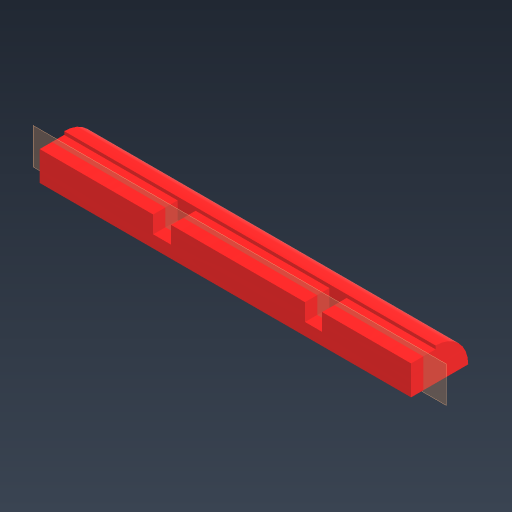
# Autodesk Inventor part: Край задней части корпуса
Saved by Autodesk Inventor 2023.2 (Build 272271030, 271C)
## iProperties
Created: 2025-04-24
Part Number: Край задней части корпуса
Material: Типовые
Document SubType Name: Modeling
Designer: Коноваленко
Density: 1 g/cm^3
Appearance: Светло-красный
Author: Коноваленко
Autodesk Inventor part; units mm, degrees
ref_plane "YZ Plane" through (0, 0, 0) normal (1, 0, 0) x (0, 1, 0)
ref_plane "XZ Plane" through (0, 0, 0) normal (0, 1, 0) x (-1, 0, 0)
ref_plane "XY Plane" through (0, 0, 0) normal (0, 0, 1) x (1, 0, 0)
sketch "Эскиз1" plane through (0, 0, 0) normal (1, 0, 0) x (0, 1, 0)
  line L0 (-8.3221, -24.9171) -> (-8.3221, 15.0829)
  line L1 (-8.3221, 15.0829) -> (31.6779, 15.0829)
  arc A0 (-8.3221, -24.9171) -> (31.6779, 15.0829) centre (-8.3221, 15.0829) ccw
  point P0 (0, 0)
  dimension "d1" = 40
  constraints: 4 end point, 2 line through centre, 2 point on circle, 1 centre point, 1 horizontal, 1 vertical
  measures "d1" distance of L0.end L1.end
extrude "Выдавливание1" add sketch "Эскиз1" along normal mid plane 455
sketch "Эскиз3" plane through (-227.5, -8.3221, 15.0829) normal (0, 0, 1) x (1, 0, 0)
  line L0 (0, 0) -> (455, 0) projected
  line L1 (455, 40) -> (455, 0) projected
  line L2 (455, 40) -> (0, 40) projected
  line L3 (0, 0) -> (0, 40) projected
  point P0 (227.5, 8.3221)
extrude "Выдавливание2" add sketch "Эскиз3" along normal blind 30
sketch "Эскиз4" plane through (-227.5, 31.6779, 15.0829) normal (0, 1, 0) x (1, 0, 0)
  line L0 (455, 0) -> (0, 0) projected
  line L1 (0, 0) -> (0, -30) projected
  line L2 (455, -30) -> (0, -30) projected
  line L3 (455, 0) -> (455, -30) projected
  point P0 (227.5, 15.0829)
extrude "Выдавливание3" cut sketch "Эскиз4" against normal blind 4
sketch "Эскиз6" plane through (-227.5, 27.6779, 15.0829) normal (0, 1, 0) x (1, 0, 0)
  line L0 (0, 40) -> (0, -30) projected
  line L1 (0, -14.536) -> (200.0528, -14.536) construction
  line L2 (455, 0) -> (0, 0) projected
  circle A0 centre (10.061, -14.536) radius 8.0645
  circle A1 centre (37.061, -14.536) radius 8.0645
  circle A2 centre (64.061, -14.536) radius 8.0645
  circle A3 centre (91.061, -14.536) radius 8.0645
  circle A4 centre (118.061, -14.536) radius 8.0645
  circle A5 centre (145.061, -14.536) radius 8.0645
  circle A6 centre (172.061, -14.536) radius 8.0645
  point P0 (227.5, 15.0829)
  dimension "d21" = 14.536
  dimension "d22" = 16.129
  dimension "d23" = 10.061
  dimension "d26" = 27
  constraints: 7 centre point, 2 end point, 2 horizontal, 2 point on line, 12 other
  measures "d21" distance between parallel lines of L2 L1
  measures "d22" diameter of A0
  measures "d23" distance from line of L0 A0.centre
  measures "d26" distance of A0.centre A1.centre
extrude "Выдавливание5" [suppressed]
sketch "Эскиз8" plane through (-227.5, -8.3221, -24.9171) normal (0, -1, 0) x (1, 0, 0)
  line L0 (455, 50) -> (465, 55)
  line L1 (465, 55) -> (465, 35)
  line L2 (465, 35) -> (455, 40)
  line L3 (455, 0) -> (455, 70) projected
  point P0 (227.5, 24.9171)
  point P1 (465, 45)
  dimension "d33" = 20
  dimension "d34" = 10
  dimension "d35" = 20
  dimension "d36" = 15
  dimension "d37" = 10
  constraints: 6 end point, 2 point on line, 1 midpoint, 1 vertical
  measures "d33" distance of L0.end L1.end
  measures "d34" distance of L2.end L0.start
  measures "d35" distance of L3.end L0.start
  measures "d36" vertical distance of L3.end L0.end
  measures "d37" distance from line of point (465, 45) L3
extrude "Выдавливание6" [suppressed]
sketch "Эскиз9" plane through (-227.5, -8.3221, -24.9171) normal (0, -1, 0) x (1, 0, 0)
  line L0 (210, 40) -> (220, 45)
  line L1 (220, 45) -> (220, 25)
  line L2 (220, 25) -> (210, 30)
  line L3 (455, 0) -> (455, 70) projected
  line L4 (-10, 25) -> (-10, 45)
  line L5 (-10, 45) -> (0, 40)
  line L6 (0, 30) -> (-10, 25)
  line L7 (0, 0) -> (0, 70) projected
  point P0 (227.5, 24.9171)
  constraints: 12 end point, 2 vertical, 13 other
extrude "Выдавливание7" [suppressed]
sketch "Эскиз10" plane through (-227.5, -8.3221, -24.9171) normal (0, -1, 0) x (1, 0, 0)
  line L0 (-10, 45) -> (0, 40)
  line L1 (-10, 25) -> (-10, 45)
  line L2 (0, 30) -> (-10, 25)
  line L3 (0, 0) -> (0, 70) projected
  point P0 (227.5, 24.9171)
  constraints: 6 end point, 1 vertical, 6 other
extrude "Выдавливание8" add sketch "Эскиз10" against normal blind 20
sketch "Эскиз11" plane through (-227.5, -8.3221, -24.9171) normal (0, -1, 0) x (1, 0, 0)
  line L0 (0, 70) -> (455, 70) projected
  line L1 (0, 0) -> (455, 0) projected
  line L2 (0, 40) -> (455, 40) projected
  point P0 (227.5, 24.9171)
feature "Разделение1" [suppressed]
sketch "Эскиз14" plane through (-227.5, 27.6779, 15.0829) normal (0, 1, 0) x (1, 0, 0)
  line L0 (0, 0) -> (455, 0) projected
  line L1 (0, -30) -> (455, -30) projected
  line L2 (134.048, 0) -> (100.336, 0)
  line L3 (100.336, 0) -> (100.336, -30) construction
  line L4 (100.336, -30) -> (134.048, -30)
  line L5 (134.048, -30) -> (134.048, 0)
  line L6 (105, 0) -> (105, -320)
  line L7 (319.048, 0) -> (285.336, 0)
  line L8 (285.336, -30) -> (319.048, -30)
  line L9 (319.048, -30) -> (319.048, 0)
  line L10 (290, 0) -> (290, -320)
  point P0 (227.5, 15.0829)
  point P1 (105, -30)
  point P2 (134.048, -30)
  point P3 (290, -30)
  point P4 (319.048, -30)
  dimension "d71" = 33.712
  dimension "d72" = 4.664
  dimension "d75" = 185
  constraints: 18 end point, 2 horizontal, 2 parallel, 2 point on line, 1 perpendicular, 1 vertical, 12 other
  measures "d71" distance between parallel lines of L3 L5
  measures "d72" distance between parallel lines of L3 L6
  measures "d75" distance of L2.start L7.start
extrude "Выдавливание10" [suppressed]
ref_plane "РабПлоскость1" through (-227.5, 31.6779, 30.0829) normal (0, 0, 1) x (1, 0, 0)
sketch "Эскиз16" plane through (-227.5, -8.3221, -24.9171) normal (0, -1, 0) x (1, 0, 0)
  circle A0 centre (115, 55) radius 2.529
  line L0 (-91, 55) -> (546, 55) construction
  line L1 (115, 360) -> (115, 40) construction
  line L2 (300, 360) -> (300, 40) construction
  circle A1 centre (300, 55) radius 2.529
  point P0 (227.5, 24.9171)
  dimension "d82" = 5.058
  constraints: 4 end point, 4 point on line, 2 centre point, 2 vertical, 1 equal radius, 4 other
  measures "d82" diameter of A0
extrude "Выдавливание11" [suppressed]
sketch "Эскиз12" plane through (-227.5, 27.6779, 15.0829) normal (0, 1, 0) x (1, 0, 0)
  line L0 (0, 0) -> (455, 0) projected
  line L1 (248.041, 0) -> (248.041, -5)
  line L2 (248.041, -5) -> (264.217, -4.95)
  line L3 (264.217, -4.95) -> (264.217, -17.926)
  line L4 (264.217, -17.926) -> (248.041, -20.945)
  line L5 (248.041, -20.945) -> (248.041, -30)
  line L6 (0, -30) -> (455, -30) projected
  line L7 (227.5, 54) -> (227.5, -44) projected
  point P0 (227.5, 15.0829)
  dimension "d54" = 20.541
  dimension "d55" = 16.176
  dimension "d56" = 12.074
  dimension "d57" = 4.95
  dimension "d58" = 9.055
  dimension "d59" = 5
  constraints: 10 end point, 4 point on line, 1 parallel, 1 perpendicular
  measures "d54" distance between parallel lines of L7 L5
  measures "d55" distance between parallel lines of L1 L3
  measures "d56" distance from line of L6 L3.end
  measures "d57" distance from line of L0 L2.end
  measures "d58" distance of L4.end L5.end
  measures "d59" distance of L1.start L1.end
feature "Разделение2" [suppressed]
sketch "Эскиз13" plane through (-227.5, 27.6779, 15.0829) normal (0, 1, 0) x (1, 0, 0)
  line L0 (0, -30) -> (455, -30) projected
  line L1 (0, 0) -> (455, 0) projected
  line L2 (346, -30) -> (324, -30)
  line L3 (324, -30) -> (324, 0)
  line L4 (324, 0) -> (346, 0)
  line L5 (346, 0) -> (346, -30)
  line L6 (325, -320) -> (325, 0)
  line L7 (161, -30) -> (139, -30)
  line L8 (139, -30) -> (139, 0)
  line L9 (139, 0) -> (161, 0)
  line L10 (161, 0) -> (161, -30)
  point P0 (227.5, 15.0829)
  point P1 (325, -30)
  point P2 (346, 0)
  point P3 (161, 0)
  dimension "d60" = 22
  dimension "d61" = 1
  dimension "d66" = 185
  constraints: 18 end point, 2 horizontal, 2 parallel, 2 point on line, 1 perpendicular, 1 vertical, 10 other
  measures "d60" distance between parallel lines of L3 L5
  measures "d61" distance between parallel lines of L3 L6
  measures "d66" distance of L2.start L7.start
extrude "Выдавливание9" cut sketch "Эскиз13" against normal blind 21 contours L8 L1 L10 L0 | L6 L1 L5 L0
sketch "Эскиз17" plane through (-227.5, -8.3221, -24.9171) normal (0, -1, 0) x (1, 0, 0)
  circle A0 centre (150, 55) radius 2.1
  line L0 (-91, 55) -> (546, 55) construction
  line L1 (150, 40) -> (150, 360) construction
  line L2 (335, 40) -> (335, 360) construction
  circle A1 centre (335, 55) radius 2.1
  point P0 (227.5, 24.9171)
  dimension "d85" = 4.2
  constraints: 4 end point, 4 point on line, 2 centre point, 2 vertical, 1 equal radius, 4 other
  measures "d85" diameter of A0
extrude "Выдавливание12" cut sketch "Эскиз17" against normal up to next
sketch "Эскиз18" plane through (-227.5, 0, 0) normal (-1, 0, 0) x (0, 0, 1)
  arc A0 (15.0829, 17.6779) -> (-10.9171, -8.3221) centre (15.0829, -8.3221) ccw
  line L0 (-24.9171, -8.3221) -> (45.0829, -8.3221) projected
  arc A1 (15.0829, 27.6779) -> (-20.9171, -8.3221) centre (15.0829, -8.3221) ccw construction
  line L1 (45.0829, 27.6779) -> (15.0829, 27.6779) projected
  line L2 (15.0829, 17.6779) -> (15.0829, 27.6779) construction
  line L3 (45.0829, -8.3221) -> (45.0829, 27.6779) projected
  arc A2 (15.6159, 17.1393) -> (-10.3841, -8.3221) centre (15.0829, -8.3221) ccw
  line L4 (15.6159, 17.1393) -> (15.6159, 28.207)
  arc A3 (15.6159, 28.207) -> (-21.4501, -8.3221) centre (15.0829, -8.3221) ccw
  point P0 (0, 0)
  point P1 (15.0829, 17.6779)
  point P2 (-21.4501, -8.3221)
  point P3 (-10.3841, -8.3221)
  dimension "d94" = 0.533
  constraints: 8 point on circle, 4 centre point, 4 end point, 1 vertical, 10 other
  measures "d94" distance between parallel lines of L4 L2
extrude "Выдавливание13" [suppressed]
sketch "Эскиз19" plane through (-227.5, 27.6779, 15.0829) normal (0, 1, 0) x (1, 0, 0)
  line L0 (237.5, 0) -> (0, 0) projected
  line L1 (105, -30) -> (0, -30) projected
  line L2 (0, 0) -> (16.614, 0)
  line L3 (16.614, 0) -> (16.614, -30)
  line L4 (16.614, -30) -> (0, -30)
  line L5 (0, -30) -> (0, 0)
  point P0 (227.5, 15.0829)
  dimension "d90" = 16.614
  constraints: 8 end point, 2 parallel, 1 horizontal, 1 perpendicular, 1 point on line
  measures "d90" distance between parallel lines of L5 L3
extrude "Выдавливание14" [suppressed]
